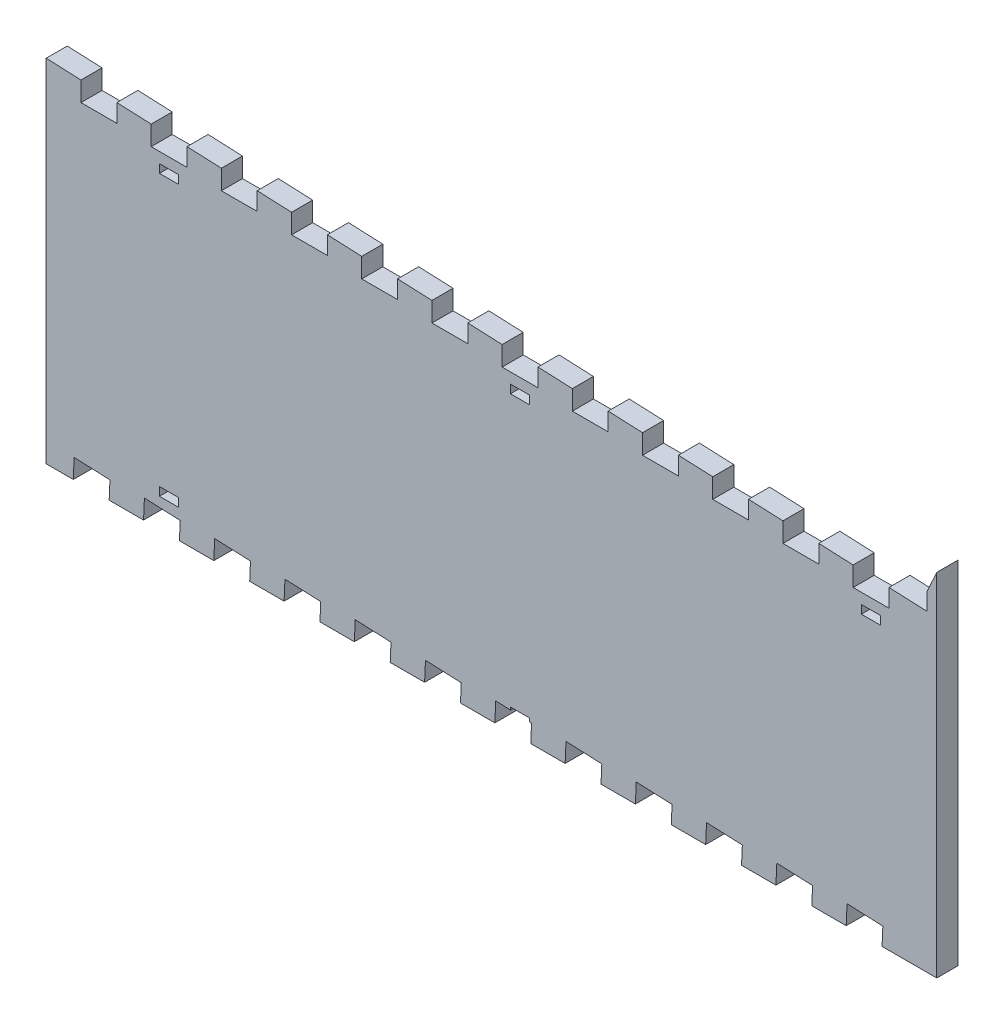
# Autodesk Inventor part: 00_Baseplate_Simmo_side3_v2
Saved by Autodesk Inventor 2024.1 (Build 281209000, 209)
## iProperties
Created: 2022-08-04
Part Number: 00_Baseplate_Simmo_side3_v2
Material: Generic
Document SubType Name: Modeling
Designer: wanghaoran
Density: 1 g/cm^3
Appearance: Default
Author: wanghaoran
Autodesk Inventor part; units mm, degrees
ref_plane "YZ Plane" through (0, 0, 0) normal (1, 0, 0) x (0, 1, 0)
ref_plane "XZ Plane" through (0, 0, 0) normal (0, 1, 0) x (-1, 0, 0)
ref_plane "XY Plane" through (0, 0, 0) normal (0, 0, 1) x (1, 0, 0)
sketch "Sketch3" plane through (0, 0, 0) normal (0, 0, 1) x (1, 0, 0)
  line L0 (0.800291, 0) -> (0.800291, 6)
  line L1 (0.800291, 0) -> (0.800291, -73)
  line L2 (-244.238532, 0) -> (-244.238532, 6)
  line L3 (0.800291, 6) -> (-249.986662, 6)
  line L4 (-249.986662, 17) -> (-249.986662, -83)
  line L5 (-249.986662, -83) -> (0.800291, -83)
  line L6 (0.800291, -83) -> (0.800291, 6)
  line L7 (-249.986662, 11) -> (-249.986662, 17)
  line L8 (3.505269, 17) -> (3.505269, -75)
  line L9 (3.505269, 11) -> (0.800291, 11)
  line L10 (0.800291, 11) -> (0.800291, -83)
  line L11 (0.800291, -83) -> (3.505269, -83)
  line L12 (3.505269, -83) -> (3.505269, 17)
  point P0 (0, 0)
  point P1 (-244.238532, 6)
  point P2 (-231.877853, 0)
  point P3 (0.800291, 4)
  dimension "d10" = 100
  constraints: 12 end point, 2 horizontal, 2 parallel, 2 vertical, 6 other
  measures "d10" distance of L4.start L4.end
sketch "Sketch3 outline for Extrusion3" plane through (0, 0, 0) normal (0, 0, 1) x (1, 0, 0)
  line L0 (0.800291, 6) -> (-249.986662, 17)
  line L1 (-249.986662, 17) -> (-249.986662, -83)
  line L2 (-249.986662, -83) -> (3.505269, -83)
  line L3 (3.505269, -83) -> (3.505269, 17)
  line L4 (3.505269, 17) -> (0.800291, 11)
  line L5 (0.800291, 11) -> (0.800291, 6)
extrude "Extrusion3" add sketch "Sketch3 outline for Extrusion3" along normal blind 6
sketch "Sketch4" plane through (0, 0, 6) normal (0, 0, 1) x (1, 0, 0)
  line L0 (0.800291, 6) -> (-249.986662, 17)
  line L1 (-229.986662, 11) -> (-229.986662, 17)
  line L2 (-239.986662, 17) -> (-229.986662, 17)
  line L3 (-239.986662, 17) -> (-239.986662, 11)
  line L4 (-239.986662, 11) -> (-229.986662, 11)
  line L5 (-229.986662, 11) -> (-229.886662, 11)
  line L6 (-229.886662, 11) -> (-229.886662, 17)
  line L7 (-229.886662, 17) -> (-229.986662, 17)
  line L8 (-229.986662, 17) -> (-229.986662, 11)
  line L9 (-239.986662, 11) -> (-240.086662, 11)
  line L10 (-240.086662, 11) -> (-240.086662, 17)
  line L11 (-240.086662, 17) -> (-239.986662, 17)
  line L12 (-239.986662, 17) -> (-239.986662, 11)
  point P0 (0, 0)
  point P1 (-249.986662, 17)
  point P2 (-229.886662, 16.118375)
  point P3 (-240.086662, 16.565767)
  dimension "d20" = 0.1
  dimension "d21" = 6
  dimension "d22" = 0.1
  dimension "d23" = 6
  constraints: 16 end point, 4 parallel, 2 horizontal, 2 perpendicular, 1 other
  measures "d20" distance of L7.end L6.end
  measures "d21" distance of L6.end L5.end
  measures "d22" distance of L10.end L11.end
  measures "d23" distance of L9.end L10.end
extrude "Extrusion4" cut sketch "Sketch4" against normal blind 6 contours L6 L5 L1 L0 | L1 L4 L3 L0 | L3 L9 L10 L0
pattern_linear "Rectangular Pattern2" count 12 spacing 20 along (0.9990395, -0.0438198, 0) of "Extrusion4"
ref_plane "Work Plane2" through (2029.894726, -83, 0) normal (-0.0219152, -0.9997598, 0) x (0, 0, -1)
mirror "Mirror2" about plane through (2029.894726, -83, 0) normal (-0.0219152, -0.9997598, 0) of "Extrusion4", "Rectangular Pattern2"
sketch "Sketch5" plane through (0, 0, 6) normal (0, 0, 1) x (1, 0, 0)
  line L0 (-212.255872, 4.723604) -> (-217.755872, 4.723604)
  line L1 (-217.755872, 4.723604) -> (-217.755872, 7.123604)
  line L2 (-217.755872, 7.123604) -> (-212.255872, 7.123604)
  line L3 (-212.255872, 7.123604) -> (-212.255872, 4.723604)
  line L4 (-209.905872, 15.241979) -> (-209.905872, 10.123604)
  line L5 (-209.905872, 10.123604) -> (-220.105872, 10.123604)
  point P0 (0, 0)
  dimension "d26" = 5.5
  dimension "d27" = 2.4
  dimension "d28" = 2.35
  dimension "d29" = 3
  constraints: 8 end point, 2 parallel, 1 horizontal, 1 perpendicular
  measures "d26" distance of L1.end L2.end
  measures "d27" distance of L0.end L1.end
  measures "d28" distance between parallel lines of L4 L3
  measures "d29" distance between parallel lines of L5 L2
extrude "Extrusion5" cut sketch "Sketch5" against normal blind 6
pattern_linear "Rectangular Pattern3" count 3 spacing 100 along (0.9990395, -0.0438198, 0) count 2 spacing 79.6 along (0, -1, 0) of "Extrusion5"
body "Solid2"
